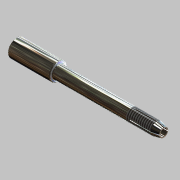
# Autodesk Inventor part: YTP-AP-E14-R1.0
Saved by Autodesk Inventor 2020.4 (Build 244396010, 396A)
## iProperties
RuleStatus: InUse
AfterDocNew0: iPropertyEnforcement
BeforeDocSave0: Materialprüfung
Created: 2021-08-29
Part Number: YTP-AP-E14-R1.0
Material: Allgemein
Document SubType Name: Modeling
Designer: Uwe Wieser
Mass: 0.343607 g
Surface Area: 8.51088 cm^2
Volume: 0.343607 cm^3
Density: 1 g/cm^3
Appearance: Chrom - poliert
Project: Airbruch
Description: Nadelmitnehmer
Werkstoff: 1.4301
Author: Uwe Wieser
Autodesk Inventor part; units mm, degrees
ref_plane "YZ Plane" through (0, 0, 0) normal (1, 0, 0) x (0, 1, 0)
ref_plane "XY Plane" through (0, 0, 0) normal (0, 0, 1) x (1, 0, 0)
sketch "Skizze1" plane through (0, 0, 0) normal (0, 0, 1) x (1, 0, 0)
  line L0 (42, 1) -> (0, 1)
  line L1 (0, 2.25) -> (0, 1)
  arc A0 (0.25, 2.5) -> (0, 2.25) centre (0.25, 2.25) ccw
  line L2 (0.25, 2.5) -> (12, 2.5)
  line L3 (12, 1.75) -> (12, 2.5)
  line L4 (34, 1) -> (34, 0.995)
  line L5 (-8.4621, 0) -> (50.4104, 0) projected
  line L6 (0, 0.6836) -> (0, 2.8631) projected
  line L7 (11.9997, 1.75) -> (39.9817, 1.75)
  line L8 (42, 1) -> (42, 1.284)
  line L9 (42, 1.284) -> (39.9817, 1.75)
  dimension "d0" = 2
  dimension "d1" = 5
  dimension "d8" = 42
  dimension "d9" = 0.25
  dimension "d10" = 3.5
  dimension "d24" = 103
  constraints: 16 end point, 3 point on line, 2 point on circle, 1 centre point, 1 parallel, 1 vertical
  measures "d0" diameter of L0 L5
  measures "d1" diameter of L2 L5
  measures "d8" distance between parallel lines of L6 L8
  measures "d9" radius of A0
  measures "d10" diameter of L7 L5
  measures "d24" angle of L9 L8
revolve "Umdrehung1" add sketch "Skizze1" angle 360 about axis through (-10, 0, 0) along (1, 0, 0)
ref_plane "Arbeitsebene1" through (0, 1.2, 0) normal (0, 1, 0) x (-1, 0, 0)
sketch "Skizze2" plane through (0, 1.2, 0) normal (0, 1, 0) x (-1, 0, 0)
  line L0 (8.4, 0) -> (-50.4, 0) projected
  arc A0 (-10.3, 1.5) -> (-10.3, -1.5) centre (-10.3, 0) ccw
  line L1 (0, 1) -> (0, -1) projected
  line L2 (-10.3, -1.5) -> (0, -1.5)
  line L3 (-42, -1) -> (0, -1) projected
  line L4 (-10.3, 1.5) -> (0, 1.5)
  line L5 (0, 2.25) -> (0, -2.25) projected
  line L6 (0, 1.5) -> (0, -1.5)
  point P0 (0, 0)
  dimension "d13" = 3
  dimension "d14" = 10.3
  constraints: 6 end point, 2 point on circle, 2 point on line, 2 tangent, 1 centre point, 1 collinear, 1 horizontal, 1 parallel
  measures "d13" diameter of A0
  measures "d14" distance from line of L1 A0.centre
extrude "Extrusion1" cut sketch "Skizze2" along normal through all
sketch "Skizze3" plane through (0, 0, 0) normal (0, 0, 1) x (1, 0, 0)
  line L0 (-8.4, 0) -> (50.4, 0) projected
  line L1 (42, 0.1) -> (34, 0.1)
  line L2 (34, 0.1) -> (34, -0.1)
  line L3 (34, -0.1) -> (42, -0.1)
  line L4 (42, -0.1) -> (42, 0.1)
  line L5 (42, -1) -> (42, 1) projected
  point P0 (0, 0)
  dimension "d17" = 8
  dimension "d18" = 0.2
  constraints: 8 end point, 2 parallel, 1 horizontal, 1 perpendicular, 1 point on line, 1 other
  measures "d17" distance of L1.start L1.end
  measures "d18" distance between parallel lines of L3 L1
extrude "Extrusion2" cut sketch "Skizze3" along normal through all both and the other way through all
pattern_circular "Runde Anordnung1" count 4 over 360 about axis through (25.9908, 0, 0) along (1, 0, 0) of "Extrusion2"
thread "Gewinde1" size "M3.5x0.6" class "6g" standard "ISO Metric profile" length 10 offset 21
fillet "Rundung1" radius 0.2 2 edges at (12, -1.75, 0) (12, -2.5, 0)
fillet "Rundung2" radius 0.1 3 edges at (11.8, 1.2, 0) (5.15, 1.2, 1.5) (5.15, 1.2, -1.5)
